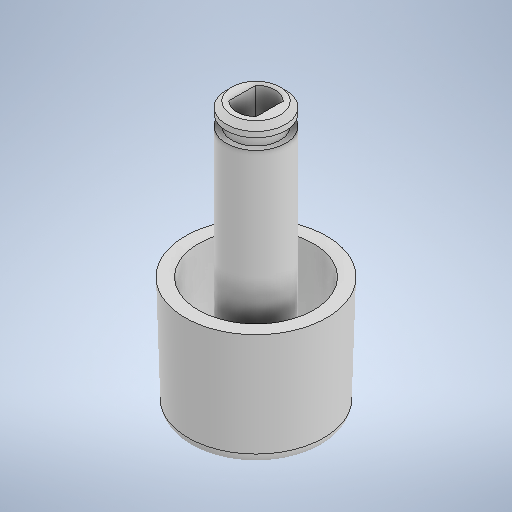
# Autodesk Inventor part: Кнопка для кухонной плиты
Saved by Autodesk Inventor 2025 (Build 290162000, 162)
## iProperties
Created: 2025-07-24
Part Number: Кнопка для кухонной плиты
Material: Типовые
Document SubType Name: Modeling
Designer: Makusimu
Density: 1 g/cm^3
Appearance: По умолчанию
Author: Makusimu
Autodesk Inventor part; units mm, degrees
ref_plane "YZ Plane" through (0, 0, 0) normal (1, 0, 0) x (0, 1, 0)
ref_plane "XZ Plane" through (0, 0, 0) normal (0, 1, 0) x (-1, 0, 0)
ref_plane "XY Plane" through (0, 0, 0) normal (0, 0, 1) x (1, 0, 0)
sketch "Эскиз1" plane through (0, 0, 0) normal (1, 0, 0) x (0, 1, 0)
  line L0 (0, 0) -> (35, 0)
  line L1 (0, 0) -> (0, 6.15)
  line L2 (0, 6.15) -> (10.5958, 6.45)
  line L3 (10.5958, 6.45) -> (10.5958, 5.25)
  line L4 (10.5958, 5.25) -> (1.2, 4.984)
  line L5 (1.2, 4.984) -> (1.2, 2.7)
  line L6 (24.5, 2.7) -> (24.5, 0)
  line L7 (22.5, 2.7) -> (22.5, 2.2)
  line L8 (22.5, 2.2) -> (23.5, 2.2)
  line L9 (23.5, 2.2) -> (23.5, 2.7)
  line L10 (24.5, 2.7) -> (23.5, 2.7)
  line L11 (22.5, 2.7) -> (1.2, 2.7)
  point P0 (0, 3.075)
  dimension "d0" = 35
  dimension "d1" = 6.15
  dimension "d2" = 10.6
  dimension "d4" = 24.5
  dimension "d5" = 2.7
  dimension "d6" = 6.45
  dimension "d7" = 1.2
  dimension "d8" = 1.2
  dimension "d11" = 1
  dimension "d12" = 1
  dimension "d21" = 0.5
  dimension "d22" = 0
  constraints: 24 end point, 3 perpendicular, 2 horizontal, 2 parallel, 2 vertical, 1 midpoint, 1 point on line
  measures "d0" distance of L0.start L0.end
  measures "d1" distance of L0.start L1.end
  measures "d2" distance of L1.end L2.end
  measures "d4" distance between parallel lines of L1 L6
  measures "d5" distance of L6.start L6.end
  measures "d6" distance from line of L0 L2.end
  measures "d7" distance of L2.end L3.end
  measures "d8" distance from line of point (0, 3.075) L5
  measures "d11" distance between parallel lines of L6 L9
  measures "d12" distance between parallel lines of L9 L7
  measures "d21" distance of L7.start L7.end
  measures "d22" vertical distance of L7.start L9.end
revolve "Вращение1" add sketch "Эскиз1" angle 360 about axis through (0, 0, 0) along (0, 1, 0)
fillet "Сопряжение1" radius 1 1 edges at (0, 0, -6.15)
sketch "Эскиз2" plane through (0, 24.5, 0) normal (0, 1, 0) x (1, 0, 0)
  circle A0 centre (0, 0) radius 1.75
  line L0 (-1.25, 1.2247) -> (-1.25, -1.2247)
  line L1 (1.25, 1.2247) -> (1.25, -1.2247)
  dimension "d13" = 3.5
  dimension "d19" = 1.25
  dimension "d20" = 1.25
  constraints: 4 end point, 4 point on circle, 1 centre point, 1 coincident, 1 vertical
  measures "d13" diameter of A0
  measures "d19" distance from line of point (0, 0) L1
  measures "d20" distance from line of point (0, 0) L0
extrude "Выдавливание1" cut sketch "Эскиз2" against normal blind 20 contours L1 A0 L0
chamfer "Фаска1" distance 0.5 angle 45 1 edges at (0, 24.5, -2.7)
